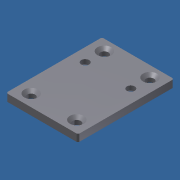
# Autodesk Inventor part: TRASEIRA DA CABINE
Saved by Autodesk Inventor 2012 SP1 (Build 160190100, 190)
## iProperties
Created: 2012-07-21
Part Number: TRASEIRA DA CABINE
Material: Carbon Steel
Document SubType Name: Modeling
Designer: BRUNO-BASSOTTI
Density: 7.87 g/cm^3
Mass: 226.656 g
Surface Area: 112.8 cm^2
Volume: 28.8 cm^3
Author: BRUNO-BASSOTTI
Autodesk Inventor part; units mm, degrees
ref_plane "YZ Plane" through (0, 0, 0) normal (1, 0, 0) x (0, 1, 0)
ref_plane "XZ Plane" through (0, 0, 0) normal (0, 1, 0) x (-1, 0, 0)
ref_plane "XY Plane" through (0, 0, 0) normal (0, 0, 1) x (1, 0, 0)
sketch "Sketch1" plane through (0, 0, 0) normal (0, 0, 1) x (1, 0, 0)
  line L0 (0, 0) -> (60, 0)
  line L1 (60, 0) -> (60, 80)
  line L2 (60, 80) -> (0, 80)
  line L3 (0, 80) -> (0, 0)
  dimension "d0" = 80
  dimension "d1" = 60
  constraints: 8 end point, 2 parallel, 1 horizontal, 1 perpendicular
  measures "d0" distance of L2.end L0.start
  measures "d1" distance of L0.start L0.end
extrude "Extrusion1" add sketch "Sketch1" along normal blind 6
sketch "Sketch2" plane through (0, 0, 6) normal (0, 0, 1) x (1, 0, 0)
  line L0 (0, 0) -> (0, 80) projected
  line L1 (60, 0) -> (0, 0) projected
  point P0 (11, 71)
  point P1 (49, 71)
  point P2 (11, 10)
  point P3 (49, 10)
  dimension "d4" = 11
  dimension "d5" = 49
  dimension "d6" = 10
  dimension "d7" = 11
  dimension "d8" = 49
  dimension "d13" = 71
  dimension "d14" = 71
  dimension "d15" = 10
  measures "d4" distance from line of L0 point (11, 71)
  measures "d5" distance from line of L0 point (49, 71)
  measures "d6" distance from line of L1 point (11, 10)
  measures "d7" distance from line of L0 point (11, 10)
  measures "d8" distance from line of L0 point (49, 10)
  measures "d13" distance from line of L1 point (11, 71)
  measures "d14" distance from line of L1 point (49, 71)
  measures "d15" distance from line of L1 point (49, 10)
hole "Hole1" at (11, 71, 6) at (49, 71, 6) at (11, 10, 6) at (49, 10, 6) direction (0, 0, -1) diameter 6.6 depth 6 tip angle 118 countersink diameter 11.5 countersink angle 90
sketch "Sketch3" plane through (0, 0, 0) normal (0, 0, -1) x (-1, 0, 0)
  line L0 (0, 0) -> (-60, 0) projected
  line L1 (-60, 0) -> (-60, 80) projected
  point P0 (-49, 55)
  point P1 (-11, 55)
  dimension "d26" = 55
  dimension "d27" = 55
  dimension "d28" = 11
  dimension "d29" = 49
  measures "d26" distance from line of L0 point (-49, 55)
  measures "d27" distance from line of L0 point (-11, 55)
  measures "d28" distance from line of L1 point (-49, 55)
  measures "d29" distance from line of L1 point (-11, 55)
hole "Hole2" at (49, 55, 0) at (11, 55, 0) direction (0, 0, 1) diameter 6.5 depth 6 tip angle 118 countersink diameter 11.5 countersink angle 90
chamfer "Chamfer2" distance 1 angle 45 4 edges at (60, 0, 3) (60, 80, 3) (0, 80, 3) (0, 0, 3)
body "Solid1"
